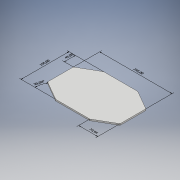
# Autodesk Inventor part: Base_petit_robot
Saved by Autodesk Inventor 2018 (Build 220112000, 112)
## iProperties
Created: 2018-01-30
Part Number: Base_petit_robot
Material: Générique
Document SubType Name: Modeling
Designer: Tristan
Density: 1 g/cm^3
Appearance: Par défaut
Author: Tristan
Autodesk Inventor part; units mm, degrees
ref_plane "YZ Plane" through (0, 0, 0) normal (1, 0, 0) x (0, 1, 0)
ref_plane "XZ Plane" through (0, 0, 0) normal (0, 1, 0) x (-1, 0, 0)
ref_plane "XY Plane" through (0, 0, 0) normal (0, 0, 1) x (1, 0, 0)
sketch "Esquisse1" plane through (0, 0, 0) normal (0, 0, 1) x (1, 0, 0)
  line L0 (0, 0) -> (295, 0)
  line L1 (295, 0) -> (295, -195)
  line L2 (295, -195) -> (0, -195)
  line L3 (0, -195) -> (0, 0)
  dimension "d0" = 295
  dimension "d1" = 195
  constraints: 8 end point, 2 parallel, 1 horizontal, 1 perpendicular
  measures "d0" distance of L0.start L0.end
  measures "d1" distance of L0.end L1.end
extrude "Extrusion1" add sketch "Esquisse1" along normal blind 6
chamfer "Chanfrein1" distance 45 angle 60 2 edges at (295, -195, 3) (295, 0, 3) measured on face at (295, -65, 2)
chamfer "Chanfrein2" distance 45 angle 60 2 edges at (0, -195, 3) (0, 0, 3) measured on face at (0, -130, 2)
